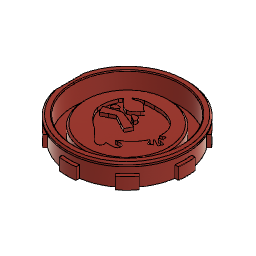
binocular-lens-covers v8 (Autodesk Fusion 360 design; units mm, degrees)
Autodesk Fusion 360 part; units mm, degrees
note: some values were not read from the file. Chosen so that the rebuilt part matches the saved one: which bodies a step acts on; which face or edge a step refers to.
sketch "Sketch1" plane through (0, 0, 0) normal (0, 0, 1) x (1, 0, 0) in component "casing"
  circle A0 centre (0, 0) radius 31.75
  circle A1 centre (0, 0) radius 33.75
  circle A2 centre (0, 0) radius 35.75
  line L0 (0, 0) -> (-35.75, 0)
  line L1 (-35.75, 0) -> (-39.75, 0)
  line L2 (-39.75, 0) -> (-39.75, -5)
  line L3 (-39.75, -5) -> (-35.75, -5)
  line L4 (-35.75, -5) -> (-35.75, 5)
  line L5 (-35.75, 5) -> (-39.75, 5)
  line L6 (-39.75, 5) -> (-39.75, 0)
  line L7 (-43.75, 0.3961) -> (-43.75, -7)
  line L8 (-34.5986, 9) -> (-41.75, 9)
  line L9 (-43.75, 7) -> (-43.75, 0.3961)
  line L10 (-41.75, -9) -> (-34.5986, -9)
  arc A3 (-43.75, -7) -> (-41.75, -9) centre (-41.75, -7) ccw
  arc A4 (-41.75, 9) -> (-43.75, 7) centre (-41.75, 7) ccw
  line L11 (-34.5986, -9) -> (-34.5986, -13) construction
  line L12 (-34.5986, -13) -> (-33.3026, -13) construction
  line L13 (-34.5986, 9) -> (-34.5986, 13) construction
  line L14 (-34.5986, 13) -> (-33.3026, 13) construction
  line L15 (-34.5986, 9) -> (-36.5986, 9) construction
  line L16 (-34.5986, -9) -> (-36.5986, -9) construction
  arc A5 (-36.5986, 9) -> (-33.3026, 13) centre (-41.0462, 16.0228) ccw construction
  arc A6 (-33.3026, -13) -> (-36.5986, -9) centre (-41.0462, -16.0228) ccw construction
  arc A7 (-33.3026, -13) -> (-36.5986, -9) centre (-41.0462, -16.0228) ccw
  arc A8 (-36.5986, 9) -> (-33.3026, 13) centre (-41.0462, 16.0228) ccw
  dimension "d1" = 63.5
  dimension "d2" = 2
  dimension "d3" = 4
  dimension "d8" = 4
  dimension "d9" = 5
  dimension "d10" = 4
  dimension "d11" = 10
  dimension "d12" = 4
  dimension "d14" = 2
  dimension "d15" = 2
  dimension "d16" = 4
  dimension "d17" = 4
  dimension "d18" = 2
  dimension "d19" = 2
  constraint coincident A0.centre A1.centre
  constraint coincident A2 L0.end
  constraint horizontal L0
  constraint parallel L0 L1
  constraint perpendicular L1 L2
  constraint perpendicular L2 L3
  constraint perpendicular L1 L4
  constraint perpendicular L4 L5
  constraint coincident A2 L8.start
  constraint coincident A2 L10.end
  constraint tangent L10 A3
  constraint tangent L7 A3
  constraint tangent L8 A4
  constraint tangent L9 A4
  constraint perpendicular L10 L11
  constraint coincident A2 L12.end
  constraint perpendicular L11 L12
  constraint perpendicular L8 L13
  constraint coincident A2 L14.end
  constraint perpendicular L13 L14
  constraint perpendicular L13 L15
  constraint perpendicular L11 L16
  constraint tangent A2 A5
  constraint tangent A2 A6
  measures "d1" diameter of A0
  measures "d8" distance of L0.end L1.end
  measures "d9" distance of L1.end L2.end
  measures "d10" distance of L2.end L3.end
  measures "d11" distance of L3.end L4.end
  measures "d12" distance of L4.end L5.end
  measures "d14" radius of A3
  measures "d15" radius of A4
  measures "d16" distance of L10.end L11.end
  measures "d17" distance of L8.start L13.end
  measures "d18" distance of L8.start L15.end
  measures "d19" distance of L10.end L16.end
extrude "Extrude1" add sketch "Sketch1" along normal blind 12 contours A2 makes body 1 in component "casing"
extrude "Extrude2" add sketch "Sketch1" against normal blind 4 contours A0 | A1 | A2 bodies 1 in component "casing"
copy_body "CutPasteBodies1" bodies 1 removing the originals makes body 2 in component "casing"
extrude "Extrude1'" add sketch "Sketch1" along normal up to surface (12 mm away) contours A2 L8 A8 | A2 L10 A7 | A2 L7 L8 L9 L10 A3 A4 bodies 2 in component "casing"
extrude "Extrude2'" add sketch "Sketch1" against normal up to surface (4 mm away) contours A2 L8 A8 | A2 L10 A7 | A2 L7 L8 L9 L10 A3 A4 bodies 2 in component "casing"
chamfer "Chamfer1" distance 1 angle 45 8 edges at (35.75, 0, -4) (-34.6309, -10.7366, -4) (-34.6309, 10.7366, -4) (-39.1743, 9, -4) (-43.1642, 8.4142, -4) (-43.75, 0, -4) (-43.1642, -8.4142, -4) (-39.1743, -9, -4) on bodies 2 in component "casing"
chamfer "Chamfer2" distance 1 angle 45 4 edges at (-35.75, 0, -4) (-37.75, 5, -4) (-39.75, 0, -4) (-37.75, -5, -4) on bodies 2 in component "casing"
chamfer "Chamfer3" distance 1 angle 45 12 edges at (-34.6309, 10.7366, 12) (35.75, 0, 12) (-34.6309, -10.7366, 12) (-39.1743, 9, 12) (-39.1743, -9, 12) (-43.1642, -8.4142, 12) (-43.75, 0, 12) (-43.1642, 8.4142, 12) (-37.75, 5, 12) (-35.75, 0, 12) (-37.75, -5, 12) (-39.75, 0, 12) on bodies 2 in component "casing"
sketch "Sketch1 (2)" plane through (0, 0, 0) normal (0, 0, 1) x (-1, 0, 0) in component "flex-seal"
  circle A0 centre (0, 0) radius 33.75
  circle A1 centre (0, 0) radius 33.75
  circle A2 centre (0, 0) radius 31.75
  dimension "d27" = 63.5
  constraint concentric A0 A1
  constraint concentric A0 A2
  measures "d27" diameter of A2
extrude "Extrude1''" add sketch "Sketch1 (2)" along normal up to surface (12 mm away) separate body makes body 3 in component "flex-seal"
ref_plane "WorkPlane1" through (0, 0, 0) normal (0, 0, 1) x (1, 0, 0) in component "casing"
ref_plane "WorkPlane2" through (0, 0, 7) normal (0, 0, 1) x (1, 0, 0) in component "casing"
split "Split1" by plane through (0, 0, 7) normal (0, 0, 1) and through (0, 0, 0) normal (0, 0, 1) bodies 2 makes body 4 at (33.708, 1.6823, 8.6667) makes body 5 at (33.5823, 3.3604, 4.6667) in component "casing"
sketch "Sketch1 (1)" plane through (0, 0, 7) normal (0, 0, 1) x (-1, 0, 0) in component "casing"
  line L0 (35.75, 5) -> (39.75, 5)
  line L1 (39.75, 5) -> (39.75, -5)
  line L2 (39.75, -5) -> (35.75, -5)
  line L3 (35.75, -5) -> (35.75, 5)
  line L4 (43.75, -7) -> (43.75, 7)
  arc A0 (43.75, 7) -> (41.75, 9) centre (41.75, 7) ccw
  line L5 (41.75, 9) -> (36.5986, 9)
  arc A1 (33.3026, 13) -> (36.5986, 9) centre (41.0462, 16.0228) ccw
  arc A2 (33.3026, 13) -> (33.3026, -13) centre (0, 0) ccw
  arc A3 (36.5986, -9) -> (33.3026, -13) centre (41.0462, -16.0228) ccw
  line L6 (36.5986, -9) -> (41.75, -9)
  arc A4 (41.75, -9) -> (43.75, -7) centre (41.75, -7) ccw
  circle A5 centre (0, 0) radius 33.75
  line L7 (0, 0) -> (0, -35.75)
  line L8 (0, 0) -> (0, 35.75)
  line L9 (0, 0) -> (43.75, 0)
  line L10 (0, 0) -> (-35.75, 0)
  line L11 (0, 0) -> (27.5045, 27.5045)
  line L12 (0, 0) -> (38.8973, 0) construction
  line L13 (0, 0) -> (-26.8158, 26.8158)
  line L14 (0, 0) -> (37.9233, 0) construction
  line L15 (0, 0) -> (30.0167, -30.0167)
  line L16 (0, 0) -> (42.45, 0) construction
  line L17 (0, 0) -> (-30.0545, -30.0545)
  line L18 (0, 0) -> (42.5035, 0) construction
  line L19 (5, 0) -> (5, 35.75)
  line L20 (-5, 0) -> (-5, 35.75)
  line L21 (3.5355, 3.5355) -> (-23.2803, 30.3514)
  line L22 (-3.5355, -3.5355) -> (-30.3514, 23.2803)
  line L23 (3.5355, -3.5355) -> (31.0401, 23.969)
  line L24 (-3.5355, 3.5355) -> (23.969, 31.0401)
  line L25 (0, -5) -> (38.8973, -5)
  line L26 (0, 5) -> (43.75, 5)
  line L27 (0, 5) -> (-35.75, 5)
  line L28 (0, -5) -> (-35.75, -5)
  line L29 (-3.5355, 3.5355) -> (-33.5901, -26.519)
  line L30 (3.5355, -3.5355) -> (-26.519, -33.5901)
  line L31 (-5, 12.0711) -> (-5, -35.75)
  line L32 (-5, 12.0711) -> (33.5522, -26.4811)
  line L33 (5, -12.0711) -> (5, -35.75)
  line L34 (5, -12.0711) -> (26.4811, -33.5522)
  dimension "d32" = 45
  dimension "d33" = 135
  dimension "d34" = 45
  dimension "d35" = 135
  dimension "d36" = 5
  dimension "d37" = -5
  dimension "d38" = 5
  dimension "d39" = -5
  dimension "d40" = 5
  dimension "d41" = -5
  dimension "d42" = 5
  dimension "d43" = -5
  dimension "d44" = 5
  dimension "d45" = -5
  dimension "d46" = 5
  dimension "d47" = -5
  dimension "d48" = 5
  dimension "d49" = -5
  constraint coincident A2.centre A5.centre
  constraint coincident A2 L7.end
  constraint vertical L7
  constraint coincident A2 L8.end
  constraint parallel L7 L8
  constraint midpoint L4 L9.end
  constraint midpoint A2 L10.end
  constraint horizontal L12
  constraint horizontal L14
  constraint horizontal L16
  constraint horizontal L18
  measures "d32" angle of L11 L12
  measures "d33" angle of L13 L14
  measures "d34" angle of L15 L16
  measures "d35" angle of L17 L18
extrude "Extrude3" cut sketch "Sketch1 (1)" against normal blind 18 contours A2 A5 L11 L23 | A2 A5 L11 L24 | A2 A5 L15 L32 | A2 A5 L15 L34 | A2 A5 L8 L19 | A2 A5 L8 L20 | A2 A5 L7 L33 | A2 A5 L7 L31 | A2 A5 L13 L21 | A2 A5 L17 L29 | A2 A5 L17 L30 | A2 A5 L10 L27 | A2 A5 L10 L28 | A2 A5 L13 L22 bodies 5 makes body 6 at (35.1571, 6.4841, 4.6667) makes body 7 at (-20.2748, -29.4448, 4.6667) makes body 8 at (20.2748, 29.4448, 2.3333) makes body 9 at (20.2748, -29.4448, 2.3333) makes body 10 at (35.1571, -6.4841, 4.6667) makes body 11 at (-28.0529, 18.7643, 4.6667) in component "casing"
sketch "Sketch2" plane through (0, 0, 0) normal (0, 0, 1) x (-1, 0, 0) in component "flex-seal"
  line L0 (39.75, -5) -> (35.75, -5)
  line L1 (35.75, -5) -> (35.75, 5)
  line L2 (35.75, 5) -> (39.75, 5)
  line L3 (39.75, 5) -> (39.75, -5)
  arc A0 (33.3026, 13) -> (33.3026, -13) centre (0, 0) ccw
  arc A1 (36.5986, -9) -> (33.3026, -13) centre (41.0462, -16.0228) ccw
  line L4 (36.5986, -9) -> (41.75, -9)
  arc A2 (41.75, -9) -> (43.75, -7) centre (41.75, -7) ccw
  line L5 (43.75, -7) -> (43.75, 7)
  arc A3 (43.75, 7) -> (41.75, 9) centre (41.75, 7) ccw
  line L6 (41.75, 9) -> (36.5986, 9)
  arc A4 (33.3026, 13) -> (36.5986, 9) centre (41.0462, 16.0228) ccw
  line L7 (35.75, 5) -> (39.75, 5)
  line L8 (39.75, 5) -> (39.75, -5)
  line L9 (39.75, -5) -> (35.75, -5)
  line L10 (35.75, -5) -> (35.75, 5)
  line L11 (27.137, -20.066) -> (28.5661, -21.4951)
  arc A5 (28.5661, -21.4951) -> (33.3026, -13) centre (0, 0) ccw
  arc A6 (36.5986, -9) -> (33.3026, -13) centre (41.0462, -16.0228) ccw
  line L12 (36.5986, -9) -> (41.75, -9)
  arc A7 (41.75, -9) -> (43.75, -7) centre (41.75, -7) ccw
  line L13 (43.75, -7) -> (43.75, 7)
  arc A8 (43.75, 7) -> (41.75, 9) centre (41.75, 7) ccw
  line L14 (41.75, 9) -> (36.5986, 9)
  arc A9 (33.3026, 13) -> (36.5986, 9) centre (41.0462, 16.0228) ccw
  arc A10 (33.3026, 13) -> (28.5661, 21.4951) centre (0, 0) ccw
  line L15 (28.5661, 21.4951) -> (27.137, 20.066)
  arc A11 (27.137, -20.066) -> (27.137, 20.066) centre (0, 0) ccw
  line L16 (20.066, 27.137) -> (21.4951, 28.5661)
  arc A12 (21.4951, 28.5661) -> (5, 35.3986) centre (0, 0) ccw
  line L17 (5, 35.3986) -> (5, 33.3776)
  arc A13 (20.066, 27.137) -> (5, 33.3776) centre (0, 0) ccw
  line L18 (-21.4951, 28.5661) -> (-20.066, 27.137)
  arc A14 (-5, 33.3776) -> (-20.066, 27.137) centre (0, 0) ccw
  line L19 (-5, 33.3776) -> (-5, 35.3986)
  arc A15 (-5, 35.3986) -> (-21.4951, 28.5661) centre (0, 0) ccw
  line L20 (-27.137, 20.066) -> (-28.5661, 21.4951)
  arc A16 (-28.5661, 21.4951) -> (-35.3986, 5) centre (0, 0) ccw
  line L21 (-35.3986, 5) -> (-33.3776, 5)
  arc A17 (-27.137, 20.066) -> (-33.3776, 5) centre (0, 0) ccw
  line L22 (-33.3776, -5) -> (-35.3986, -5)
  arc A18 (-35.3986, -5) -> (-28.5661, -21.4951) centre (0, 0) ccw
  line L23 (-28.5661, -21.4951) -> (-27.137, -20.066)
  arc A19 (-33.3776, -5) -> (-27.137, -20.066) centre (0, 0) ccw
  line L24 (-5, -35.3986) -> (-5, -33.3776)
  arc A20 (-20.066, -27.137) -> (-5, -33.3776) centre (0, 0) ccw
  line L25 (-20.066, -27.137) -> (-21.4951, -28.5661)
  arc A21 (-21.4951, -28.5661) -> (-5, -35.3986) centre (0, 0) ccw
  line L26 (21.4951, -28.5661) -> (20.066, -27.137)
  arc A22 (5, -33.3776) -> (20.066, -27.137) centre (0, 0) ccw
  line L27 (5, -33.3776) -> (5, -35.3986)
  arc A23 (5, -35.3986) -> (21.4951, -28.5661) centre (0, 0) ccw
  circle A24 centre (0, 0) radius 33.75
  circle A25 centre (0, 0) radius 33.75
extrude "Extrude2''" add sketch "Sketch2" along normal up to surface (7 mm away) contours A0 L15 L16 A24 A25 | A0 L17 L19 A24 A25 | A0 L11 L26 A24 A25 | A0 L18 L20 A24 A25 | A0 L24 L27 A24 A25 | A0 L21 L22 A24 A25 | A0 L23 L25 A24 A25 bodies 3 in component "flex-seal"
chamfer "Chamfer1'" distance 1 angle 45 1 edges at (29.6014, 11.4813, 12) on bodies 3 in component "flex-seal"
sketch "Sketch3" plane through (0, 0, 0) normal (0, 0, 1) x (-1, 0, 0) in component "flex-seal"
  line L0 (39.75, -5) -> (35.75, -5)
  line L1 (35.75, -5) -> (35.75, 5)
  line L2 (35.75, 5) -> (39.75, 5)
  line L3 (39.75, 5) -> (39.75, -5)
  arc A0 (33.3026, 13) -> (33.3026, -13) centre (0, 0) ccw
  arc A1 (36.5986, -9) -> (33.3026, -13) centre (41.0462, -16.0228) ccw
  line L4 (36.5986, -9) -> (41.75, -9)
  arc A2 (41.75, -9) -> (43.75, -7) centre (41.75, -7) ccw
  line L5 (43.75, -7) -> (43.75, 7)
  arc A3 (43.75, 7) -> (41.75, 9) centre (41.75, 7) ccw
  line L6 (41.75, 9) -> (36.5986, 9)
  arc A4 (33.3026, 13) -> (36.5986, 9) centre (41.0462, 16.0228) ccw
  circle A5 centre (0, 0) radius 31.75
extrude "Extrude3'" add sketch "Sketch3" along normal blind 2 contours A5 bodies 3 in component "flex-seal"
fillet "Fillet1" radius 1 1 edges at (29.6014, -11.4813, 2) on bodies 3 in component "flex-seal"
sketch "Sketch4" plane through (0, 0, 2) normal (0, 0, 1) x (-1, 0, 0) in component "flex-seal"
  circle A0 centre (0, 0) radius 30.75
  circle A1 centre (0, 0) radius 25.5
  dimension "d59" = 51
  constraint concentric A0 A1
  measures "d59" diameter of A1
extrude "Extrude4" add sketch "Sketch4" along normal blind 7 contours A1 bodies 3 in component "flex-seal"
chamfer "Chamfer2'" distance 1 angle 45 1 edges at (23.7743, 9.2212, 9) on bodies 3 in component "flex-seal"
sketch "Sketch5" plane through (0, 0, 9) normal (0, 0, 1) x (-1, 0, 0) in component "flex-seal"
  circle A0 centre (0, 0) radius 24.5
  spline S0 degree 3 poles (-2.8738, 19.1652) (-3.9223, 18.2735) (-4.1101, 17.1626) (-3.3274, 16.4272) knots 0 0 0 0 1 1 1 1
  spline S1 degree 3 poles (-3.3274, 16.4272) (-3.0456, 16.1768) (-2.8579, 15.9263) (-2.9052, 15.8954) knots 0 0 0 0 1 1 1 1
  spline S2 degree 3 poles (-2.9052, 15.8954) (-2.952, 15.8486) (-3.5624, 15.8954) (-4.2978, 15.9895) knots 0 0 0 0 1 1 1 1
  spline S3 degree 3 poles (-4.2978, 15.9895) (-5.6745, 16.1772) (-7.568, 16.099) (-8.538, 15.8172) knots 0 0 0 0 1 1 1 1
  spline S4 degree 3 poles (-8.538, 15.8172) (-8.8511, 15.7231) (-9.3361, 15.4259) (-9.6175, 15.16) knots 0 0 0 0 1 1 1 1
  spline S5 degree 3 poles (-9.6175, 15.16) (-10.0711, 14.7064) (-10.1025, 14.5968) (-10.0398, 13.7987) knots 0 0 0 0 1 1 1 1
  spline S6 degree 3 poles (-10.0398, 13.7987) (-9.9771, 13.126) (-9.8834, 12.8756) (-9.5389, 12.5938) knots 0 0 0 0 1 1 1 1
  spline S7 degree 3 poles (-9.5389, 12.5938) (-8.8349, 11.9834) (-7.9899, 11.8429) (-6.425, 12.062) knots 0 0 0 0 1 1 1 1
  spline S8 degree 3 poles (-6.425, 12.062) (-5.2515, 12.2183) (-4.657, 12.2029) (-4.9229, 12.0151) knots 0 0 0 0 1 1 1 1
  spline S9 degree 3 poles (-4.9229, 12.0151) (-4.9542, 11.9838) (-5.8305, 11.4048) (-6.8632, 10.732) knots 0 0 0 0 1 1 1 1
  spline S10 degree 3 poles (-6.8632, 10.732) (-10.1334, 8.5727) (-13.216, 5.1774) (-14.5459, 2.2826) knots 0 0 0 0 1 1 1 1
  spline S11 degree 3 poles (-14.5459, 2.2826) (-14.765, 1.8131) (-14.9995, 1.4222) (-15.0467, 1.4222) knots 0 0 0 0 1 1 1 1
  spline S12 degree 3 poles (-15.0467, 1.4222) (-15.1095, 1.4376) (-15.4222, 2.0167) (-15.7508, 2.7366) knots 0 0 0 0 1 1 1 1
  spline S13 degree 3 poles (-15.7508, 2.7366) (-16.0794, 3.4407) (-16.408, 4.1138) (-16.4862, 4.2388) knots 0 0 0 0 1 1 1 1
  spline S14 degree 3 poles (-16.4862, 4.2388) (-16.5803, 4.3951) (-16.8462, 4.2701) (-17.5657, 3.7693) knots 0 0 0 0 1 1 1 1
  line L0 (-17.5657, 3.7693) -> (-18.5357, 3.0966)
  line L1 (-18.5357, 3.0966) -> (-18.1602, 2.6898)
  spline S15 degree 3 poles (-18.1602, 2.6898) (-15.4377, -0.33) (-15.4531, -0.3769) (-18.5202, 1.2817) knots 0 0 0 0 1 1 1 1
  spline S16 degree 3 poles (-18.5202, 1.2817) (-19.6469, 1.8921) (-20.6169, 2.3457) (-20.6637, 2.2989) knots 0 0 0 0 1 1 1 1
  spline S17 degree 3 poles (-20.6637, 2.2989) (-20.7264, 2.252) (-20.9455, 1.6571) (-21.1801, 0.9844) knots 0 0 0 0 1 1 1 1
  line L2 (-21.1801, 0.9844) -> (-21.6031, -0.2372)
  line L3 (-21.6031, -0.2372) -> (-19.1933, -0.8472)
  spline S18 degree 3 poles (-19.1933, -0.8472) (-17.8788, -1.1758) (-16.7993, -1.5358) (-16.7993, -1.6294) knots 0 0 0 0 1 1 1 1
  spline S19 degree 3 poles (-16.7993, -1.6294) (-16.7993, -1.7235) (-17.3002, -1.9735) (-17.9102, -2.1771) knots 0 0 0 0 1 1 1 1
  spline S20 degree 3 poles (-17.9102, -2.1771) (-18.5206, -2.3962) (-19.0369, -2.5998) (-19.0524, -2.6466) knots 0 0 0 0 1 1 1 1
  spline S21 degree 3 poles (-19.0524, -2.6466) (-19.0838, -2.6934) (-18.9429, -3.1629) (-18.7551, -3.7106) knots 0 0 0 0 1 1 1 1
  line L4 (-18.7551, -3.7106) -> (-18.3952, -4.6965)
  line L5 (-18.3952, -4.6965) -> (-17.378, -3.836)
  spline S22 degree 3 poles (-17.378, -3.836) (-16.8148, -3.3511) (-16.2826, -2.9597) (-16.2044, -2.9597) knots 0 0 0 0 1 1 1 1
  spline S23 degree 3 poles (-16.2044, -2.9597) (-16.1262, -2.9597) (-16.0167, -3.8984) (-15.9699, -5.0251) knots 0 0 0 0 1 1 1 1
  spline S24 degree 3 poles (-15.9699, -5.0251) (-15.8758, -7.419) (-15.6258, -8.4517) (-14.7181, -10.3138) knots 0 0 0 0 1 1 1 1
  spline S25 degree 3 poles (-14.7181, -10.3138) (-14.2018, -11.3937) (-13.8264, -11.8942) (-12.731, -12.9737) knots 0 0 0 0 1 1 1 1
  spline S26 degree 3 poles (-12.731, -12.9737) (-11.1661, -14.5227) (-9.6643, -15.4458) (-7.4422, -16.1971) knots 0 0 0 0 1 1 1 1
  spline S27 degree 3 poles (-7.4422, -16.1971) (-4.5943, -17.1671) (-3.7184, -17.2766) (0.8818, -17.2766) knots 0 0 0 0 1 1 1 1
  spline S28 degree 3 poles (0.8818, -17.2766) (4.5902, -17.2611) (5.2006, -17.2298) (6.6401, -16.9166) knots 0 0 0 0 1 1 1 1
  spline S29 degree 3 poles (6.6401, -16.9166) (8.6272, -16.4785) (9.9417, -15.9622) (10.9744, -15.2113) knots 0 0 0 0 1 1 1 1
  line L6 (10.9744, -15.2113) -> (11.7566, -14.6481)
  line L7 (11.7566, -14.6481) -> (10.9585, -14.429)
  spline S30 degree 3 poles (10.9585, -14.429) (10.1762, -14.21) (10.1604, -14.21) (9.3472, -14.7108) knots 0 0 0 0 1 1 1 1
  spline S31 degree 3 poles (9.3472, -14.7108) (8.6586, -15.1331) (8.3145, -15.2426) (7.4537, -15.2895) knots 0 0 0 0 1 1 1 1
  spline S32 degree 3 poles (7.4537, -15.2895) (6.8592, -15.3208) (6.1392, -15.274) (5.8265, -15.1644) knots 0 0 0 0 1 1 1 1
  spline S33 degree 3 poles (5.8265, -15.1644) (5.1224, -14.9299) (3.933, -13.8659) (3.2289, -12.8332) knots 0 0 0 0 1 1 1 1
  spline S34 degree 3 poles (3.2289, -12.8332) (2.8063, -12.2073) (2.5408, -11.9883) (2.0554, -11.8474) knots 0 0 0 0 1 1 1 1
  spline S35 degree 3 poles (2.0554, -11.8474) (0.9441, -11.5346) (0.9287, -11.4406) (1.9772, -10.2043) knots 0 0 0 0 1 1 1 1
  spline S36 degree 3 poles (1.9772, -10.2043) (3.7925, -8.0294) (5.6542, -6.809) (7.1405, -6.809) knots 0 0 0 0 1 1 1 1
  spline S37 degree 3 poles (7.1405, -6.809) (8.7054, -6.809) (10.8644, -8.2485) (12.9925, -10.7365) knots 0 0 0 0 1 1 1 1
  line L8 (12.9925, -10.7365) -> (14.1033, -12.0351)
  line L9 (14.1033, -12.0351) -> (14.3692, -11.6751)
  spline S38 degree 3 poles (14.3692, -11.6751) (14.5256, -11.4874) (14.9324, -10.7988) (15.261, -10.1416) knots 0 0 0 0 1 1 1 1
  spline S39 degree 3 poles (15.261, -10.1416) (16.9668, -6.9027) (17.6863, -2.7407) (17.0763, 0.4359) knots 0 0 0 0 1 1 1 1
  spline S40 degree 3 poles (17.0763, 0.4359) (16.3877, 4.0348) (12.8516, 8.3845) (7.9228, 11.7016) knots 0 0 0 0 1 1 1 1
  spline S41 degree 3 poles (7.9228, 11.7016) (7.0624, 12.2807) (6.4051, 12.9065) (5.5288, 13.9705) knots 0 0 0 0 1 1 1 1
  spline S42 degree 3 poles (5.5288, 13.9705) (3.8389, 16.0518) (1.3196, 18.4457) (0.146, 19.0716) knots 0 0 0 0 1 1 1 1
  spline S43 degree 3 poles (0.146, 19.0716) (-1.1057, 19.7288) (-2.1539, 19.7602) (-2.8738, 19.1652) knots 0 0 0 0 1 1 1 1
  line L10 (3.0254, 1.1245) -> (7.3751, -1.2067)
  line L11 (7.3751, -1.2067) -> (10.7235, 0.4986)
  spline S44 degree 3 poles (10.7235, 0.4986) (12.5543, 1.4376) (14.1502, 2.2044) (14.2597, 2.2044) knots 0 0 0 0 1 1 1 1
  spline S45 degree 3 poles (14.2597, 2.2044) (14.3538, 2.2044) (14.8074, 1.4063) (15.261, 0.4204) knots 0 0 0 0 1 1 1 1
  spline S46 degree 3 poles (15.261, 0.4204) (15.9809, -1.1599) (16.1687, -1.7076) (16.0123, -1.7076) knots 0 0 0 0 1 1 1 1
  spline S47 degree 3 poles (16.0123, -1.7076) (15.9809, -1.7076) (14.651, -2.1616) (13.0707, -2.7089) knots 0 0 0 0 1 1 1 1
  spline S48 degree 3 poles (13.0707, -2.7089) (11.4748, -3.2566) (9.5035, -3.898) (8.6741, -4.1325) knots 0 0 0 0 1 1 1 1
  line L12 (8.6741, -4.1325) -> (7.1564, -4.5552)
  line L13 (7.1564, -4.5552) -> (5.7011, -4.0075)
  spline S49 degree 3 poles (5.7011, -4.0075) (2.0086, -2.5835) (-3.3897, -0.4555) (-3.4679, -0.3773) knots 0 0 0 0 1 1 1 1
  spline S50 degree 3 poles (-3.4679, -0.3773) (-3.562, -0.2836) (-1.6217, 3.4561) (-1.4653, 3.4561) knots 0 0 0 0 1 1 1 1
  spline S51 degree 3 poles (-1.4653, 3.4561) (-1.3871, 3.4557) (0.6314, 2.4076) (3.0254, 1.1245) knots 0 0 0 0 1 1 1 1
  spline S52 degree 3 poles (1.3823, -4.3833) (2.3995, -5.0092) (3.2286, -5.5882) (3.2286, -5.6819) knots 0 0 0 0 1 1 1 1
  spline S53 degree 3 poles (3.2286, -5.6819) (3.2286, -6.386) (1.7736, -7.1372) (0.8032, -6.965) knots 0 0 0 0 1 1 1 1
  spline S54 degree 3 poles (0.8032, -6.965) (0.0524, -6.8241) (-0.7926, -6.0419) (-0.9803, -5.3378) knots 0 0 0 0 1 1 1 1
  spline S55 degree 3 poles (-0.9803, -5.3378) (-1.1839, -4.6024) (-0.9021, -3.2725) (-0.558, -3.2725) knots 0 0 0 0 1 1 1 1
  spline S56 degree 3 poles (-0.558, -3.2725) (-0.4953, -3.2725) (0.381, -3.7733) (1.3823, -4.3833) knots 0 0 0 0 1 1 1 1
  spline S57 degree 3 poles (13.8374, -3.742) (13.9628, -3.9765) (14.0093, -4.446) (13.9783, -4.9001) knots 0 0 0 0 1 1 1 1
  spline S58 degree 3 poles (13.9783, -4.9001) (13.9156, -5.5573) (13.8219, -5.7605) (13.337, -6.1986) knots 0 0 0 0 1 1 1 1
  spline S59 degree 3 poles (13.337, -6.1986) (12.852, -6.6368) (12.6639, -6.715) (11.9912, -6.715) knots 0 0 0 0 1 1 1 1
  spline S60 degree 3 poles (11.9912, -6.715) (11.553, -6.715) (10.9898, -6.6054) (10.7394, -6.4804) knots 0 0 0 0 1 1 1 1
  spline S61 degree 3 poles (10.7394, -6.4804) (10.1917, -6.1986) (9.8631, -5.6513) (10.0822, -5.4319) knots 0 0 0 0 1 1 1 1
  spline S62 degree 3 poles (10.0822, -5.4319) (10.5049, -5.0096) (13.1961, -3.2884) (13.3993, -3.3197) knots 0 0 0 0 1 1 1 1
  spline S63 degree 3 poles (13.3993, -3.3197) (13.5243, -3.3352) (13.712, -3.5229) (13.8374, -3.742) knots 0 0 0 0 1 1 1 1
extrude "Extrude5" cut sketch "Sketch5" against normal blind 2 contours S0 S1 S2 S3 S4 S5 S6 S7 S8 S9 S10 S11 S12 S13 S14 L0 L1 S15 S16 S17 L2 L3 S18 S19 S20 S21 L4 L5 S22 S23 S24 S25 S26 S27 S28 S29 L6 L7 S30 S31 S32 S33 S34 S35 S36 S37 L8 L9 S38 S39 S40 S41 S42 S43 bodies 3 in component "flex-seal"
delete_face "DeleteFace1" 1 faces at (-32.3764, 1.6158, 11.6667) on bodies 3 in component "flex-seal"
delete_face "DeleteFace2" 1 faces at (-24.3013, -20.3912, 2.7694) on bodies 3 in component "flex-seal"
extrude "Extrude6" add 1 faces at (-32.8395, 3.2541, 12) along direction (0, 0, 1) blind 2 on bodies 3 bodies 3 in component "flex-seal"
sketch "Sketch2 (2)" plane through (0, 0, 14) normal (0, 0, 1) x (-1, 0, 0)
  circle A0 centre (0, 0) radius 31.75
  circle A1 centre (0, 0) radius 33.75
  circle A2 centre (0, 0) radius 35.75
  dimension "d67" = 2
extrude "Extrude7" add sketch "Sketch2 (2)" against normal blind 2 contours A2 bodies 3 in component "flex-seal"
chamfer "Chamfer3'" distance 1 angle 45 1 edges at (33.3307, 12.9278, 14) on bodies 3 in component "flex-seal"
chamfer "Chamfer4" distance 0.5 angle 45 1 edges at (29.6014, -11.4813, 14) on bodies 3 in component "flex-seal"
sketch "Sketch3 (2)" plane through (0, 0, 12) normal (0, 0, -1) x (1, 0, 0)
  circle A0 centre (0, 0) radius 33.75
  circle A1 centre (0, 0) radius 35.75
  line L0 (-34.75, -6) -> (-34.75, 6)
  line L1 (-34.75, -6) -> (-34.75, 6)
  line L2 (-34.75, 6) -> (-34.75, 12.16)
  line L3 (-34.75, 12.16) -> (-34.75, -15.5)
  constraint coincident L0.start L1.start
  constraint coincident L0.end L1.end
  constraint parallel L1 L2
  constraint parallel L1 L3
extrude "Extrude8" cut sketch "Sketch3 (2)" against normal blind 3 contours A1 L0 L1 L2 L3 picked at (-35.0833, 0) bodies 3 in component "flex-seal"
delete_face "DeleteFace3" 1 faces at (34.9855, -2.618, 13.6667) on bodies 3 in component "flex-seal"
chamfer "Chamfer5" distance 1 angle 45 2 edges at (35.75, 0, 14) (-34.75, 0, 14) on bodies 3 in component "flex-seal"
component "casing" placed x (1, 0, 0) y (0, 1, 0) z (0, 0, 1) at (0, 0, 0)
component "flex-seal" placed x (1, 0, 0) y (0, 1, 0) z (0, 0, 1) at (0, 0, 0)
